Autodesk Inventor part; units mm, degrees
note: some values were not read from the file. Chosen so that the rebuilt part matches the saved one: direction of "Hole2".
(part 13 of 20)
  line L1144 (-97.751541, -32.701603) -> (-97.575214, -32.525276)
  line L1145 (-97.575214, -32.525276) -> (-96.427868, -32.525276)
  line L1146 (-96.251541, -32.701603) -> (-96.427868, -32.525276)
  line L1147 (-96.427868, -32.525276) -> (-96.427868, -31.87793)
  circle A26 centre (-97.263452, -32.201603) radius 0.1
  line L1148 (-97.101541, -32.351603) -> (-97.425364, -32.351603)
  line L1149 (-97.425364, -32.351603) -> (-97.425364, -32.051603)
  line L1150 (-97.425364, -32.051603) -> (-97.101541, -32.051603)
  line L1151 (-97.101541, -32.051603) -> (-97.101541, -32.351603)
  line L1152 (-98.151541, -33.912275) -> (-97.951541, -33.912275)
  line L1153 (-97.951541, -33.912275) -> (-97.951541, -34.160588)
  line L1154 (-98.151541, -33.912275) -> (-98.151541, -33.451603)
  line L1155 (-96.051541, -34.160588) -> (-97.951541, -34.160588)
  line L1156 (-95.851541, -33.451603) -> (-95.851541, -33.912275)
  line L1157 (-96.051541, -34.160588) -> (-96.051541, -33.912275)
  line L1158 (-96.051541, -33.912275) -> (-95.851541, -33.912275)
  line L1159 (-96.251541, -33.451603) -> (-96.251541, -33.912275)
  line L1160 (-96.251541, -33.912275) -> (-97.751541, -33.912275)
  line L1161 (-97.751541, -33.912275) -> (-97.751541, -33.451603)
  line L1162 (-97.575214, -33.451603) -> (-97.575214, -33.621159)
  line L1163 (-97.751541, -33.912275) -> (-97.575214, -33.621159)
  line L1164 (-97.575214, -33.621159) -> (-96.427868, -33.621159)
  line L1165 (-96.251541, -33.912275) -> (-96.427868, -33.621159)
  line L1166 (-96.427868, -33.621159) -> (-96.427868, -33.451603)
  line L1167 (-97.101541, -33.471854) -> (-97.425364, -33.471854)
  line L1168 (-97.425364, -33.471854) -> (-97.425364, -33.451603)
  line L1169 (-97.101541, -33.451603) -> (-97.101541, -33.471854)
  line L1170 (-105.474058, -21.298) -> (-105.497268, -21.496648)
  line L1171 (-105.474199, -21.298054) -> (-105.474058, -21.298)
  line L1172 (-105.745579, -21.467637) -> (-105.74572, -21.467691)
  line L1173 (-105.497268, -21.496648) -> (-105.745579, -21.467637)
  line L1174 (-105.713438, -23.585748) -> (-105.741108, -23.582515)
  line L1175 (-105.96621, -23.354854) -> (-105.74572, -21.467691)
  line L1176 (-105.474058, -21.298) -> (-105.214117, -21.32837)
  line L1177 (-104.271292, -21.775052) -> (-104.476203, -23.528871)
  line L1178 (-105.966068, -23.3548) -> (-105.745579, -21.467637)
  line L1179 (-104.747723, -23.698507) -> (-105.740967, -23.58246)
  line L1180 (-105.741108, -23.582515) -> (-105.729814, -23.485843)
  line L1181 (-105.745774, -23.380609) -> (-105.96621, -23.354854)
  line L1182 (-105.966068, -23.3548) -> (-105.717757, -23.383811)
  line L1183 (-105.717757, -23.383811) -> (-105.740967, -23.58246)
  line L1184 (-105.740967, -23.58246) -> (-105.741108, -23.582515)
  line L1185 (-105.717757, -23.383811) -> (-105.717899, -23.383866)
  line L1186 (-105.96621, -23.354854) -> (-105.966068, -23.3548)
  line L1187 (-104.476203, -23.528871) -> (-104.476344, -23.528925)
  line L1188 (-104.747723, -23.698507) -> (-104.724514, -23.499859)
  line L1189 (-104.724514, -23.499859) -> (-104.476203, -23.528871)
  line L1190 (-104.747864, -23.698562) -> (-104.747723, -23.698507)
  line L1191 (-104.527233, -21.811344) -> (-104.701304, -23.30121)
  line L1192 (-104.701304, -23.30121) -> (-105.694548, -23.185163)
  line L1193 (-105.694548, -23.185163) -> (-105.520477, -21.695297)
  line L1194 (-105.520477, -21.695297) -> (-104.527233, -21.811344)
  line L1195 (-104.856079, -23.105651) -> (-104.722932, -21.966057)
  line L1196 (-104.701304, -23.30121) -> (-104.856079, -23.105651)
  line L1197 (-104.527233, -21.811344) -> (-104.722932, -21.966057)
  line L1198 (-104.722932, -21.966057) -> (-105.365905, -21.890934)
  line L1199 (-105.520477, -21.695297) -> (-105.365905, -21.890934)
  line L1200 (-105.365905, -21.890934) -> (-105.499051, -23.030528)
  line L1201 (-105.694548, -23.185163) -> (-105.499051, -23.030528)
  line L1202 (-105.499051, -23.030528) -> (-104.856079, -23.105651)
  circle A27 centre (-105.080572, -22.238141) radius 0.1
  line L1203 (-105.248353, -22.381553) -> (-105.210775, -22.059918)
  line L1204 (-105.210795, -22.059926) -> (-105.210775, -22.059918)
  line L1205 (-105.248374, -22.381561) -> (-105.210795, -22.059926)
  line L1206 (-105.248374, -22.381561) -> (-105.248353, -22.381553)
  line L1207 (-105.210775, -22.059918) -> (-104.912801, -22.094733)
  line L1208 (-104.912801, -22.094733) -> (-104.95038, -22.416367)
  line L1209 (-104.9504, -22.416375) -> (-104.95038, -22.416367)
  line L1210 (-104.95038, -22.416367) -> (-105.248353, -22.381553)
  line L1211 (-104.9504, -22.416375) -> (-105.248374, -22.381561)
  line L1212 (-104.238991, -32.139646) -> (-104.43764, -32.116436)
  line L1213 (-104.238849, -32.139591) -> (-104.238991, -32.139646)
  line L1214 (-104.437498, -32.116382) -> (-104.238849, -32.139591)
  line L1215 (-104.43764, -32.116436) -> (-104.437498, -32.116382)
  line L1216 (-104.268003, -32.387957) -> (-104.238991, -32.139646)
  line L1217 (-104.267861, -32.387902) -> (-104.268003, -32.387957)
  line L1218 (-104.238849, -32.139591) -> (-104.267861, -32.387902)
  line L1219 (-104.122936, -31.146332) -> (-104.096258, -30.918)
  line L1220 (-104.321451, -31.123138) -> (-104.321593, -31.123193)
  line L1221 (-104.122802, -31.146348) -> (-104.321451, -31.123138)
  line L1222 (-104.09379, -30.898037) -> (-104.122802, -31.146348)
  line L1223 (-104.093932, -30.898091) -> (-104.09379, -30.898037)
  line L1224 (-104.43764, -32.116436) -> (-104.321593, -31.123193)
  line L1225 (-102.38084, -32.608447) -> (-104.268003, -32.387957)
  line L1226 (-104.437498, -32.116382) -> (-104.321451, -31.123138)
  line L1227 (-104.09379, -30.898037) -> (-102.206627, -31.118527)
  line L1228 (-102.380698, -32.608392) -> (-104.267861, -32.387902)
  line L1229 (-102.03699, -31.390047) -> (-102.153038, -32.383291)
  line L1230 (-102.153179, -32.383345) -> (-102.351695, -32.360151)
  line L1231 (-102.380698, -32.608392) -> (-102.351686, -32.360081)
  line L1232 (-102.351686, -32.360081) -> (-102.153038, -32.383291)
  line L1233 (-102.153038, -32.383291) -> (-102.153179, -32.383345)
  line L1234 (-102.38084, -32.608447) -> (-102.380698, -32.608392)
  line L1235 (-102.03699, -31.390047) -> (-102.235639, -31.366837)
  line L1236 (-102.235639, -31.366837) -> (-102.206627, -31.118527)
  line L1237 (-103.924153, -31.169557) -> (-102.434288, -31.343628)
  line L1238 (-102.434288, -31.343628) -> (-102.550335, -32.336872)
  line L1239 (-102.550335, -32.336872) -> (-104.040201, -32.162801)
  line L1240 (-104.040201, -32.162801) -> (-103.924153, -31.169557)
  line L1241 (-102.629987, -31.49834) -> (-103.769581, -31.365194)
  line L1242 (-102.434288, -31.343628) -> (-102.629987, -31.49834)
  line L1243 (-103.924153, -31.169557) -> (-103.769581, -31.365194)
  line L1244 (-103.769581, -31.365194) -> (-103.844704, -32.008166)
  line L1245 (-104.040201, -32.162801) -> (-103.844704, -32.008166)
  line L1246 (-103.844704, -32.008166) -> (-102.70511, -32.141313)
  line L1247 (-102.550335, -32.336872) -> (-102.70511, -32.141313)
  line L1248 (-102.70511, -32.141313) -> (-102.629987, -31.49834)
  circle A28 centre (-103.497462, -31.72285) radius 0.1
  line L1249 (-103.354057, -31.890627) -> (-103.675692, -31.853049)
  line L1250 (-103.675712, -31.853056) -> (-103.675692, -31.853049)
  line L1251 (-103.354077, -31.890635) -> (-103.675712, -31.853056)
  line L1252 (-103.354077, -31.890635) -> (-103.354057, -31.890627)
  line L1253 (-103.675692, -31.853049) -> (-103.640877, -31.555076)
  line L1254 (-103.640898, -31.555083) -> (-103.640877, -31.555076)
  line L1255 (-103.675712, -31.853056) -> (-103.640898, -31.555083)
  line L1256 (-103.640877, -31.555076) -> (-103.319243, -31.592654)
  line L1257 (-103.319243, -31.592654) -> (-103.354057, -31.890627)
  line L1258 (-100.436541, -20.036387) -> (-100.436541, -20.235039)
  line L1259 (-100.436541, -20.235039) -> (-100.686541, -20.235039)
  line L1260 (-99.436541, -20.235039) -> (-99.436541, -20.036387)
  line L1261 (-99.186541, -20.235039) -> (-99.436541, -20.235039)
  line L1262 (-99.186541, -22.284516) -> (-99.436541, -22.284516)
  line L1263 (-99.186541, -22.12223) -> (-99.186541, -22.284516)
  line L1264 (-99.436541, -22.320882) -> (-99.436541, -22.12223)
  line L1265 (-99.436541, -22.12223) -> (-99.186541, -22.12223)
  line L1266 (-99.436541, -22.483167) -> (-99.436541, -22.320882)
  line L1267 (-99.436541, -22.483167) -> (-100.436541, -22.483167)
  line L1268 (-100.436541, -20.036387) -> (-99.436541, -20.036387)
  line L1269 (-99.186541, -20.235039) -> (-99.186541, -22.12223)
  line L1270 (-100.686541, -22.12223) -> (-100.686541, -20.235039)
  line L1271 (-99.436541, -22.320882) -> (-100.436541, -22.320882)
  line L1272 (-100.436541, -22.284516) -> (-100.686541, -22.284516)
  line L1273 (-100.686541, -22.12223) -> (-100.436541, -22.12223)
  line L1274 (-100.436541, -22.12223) -> (-100.436541, -22.320882)
  line L1275 (-100.436541, -22.320882) -> (-100.436541, -22.483167)
  line L1276 (-100.686541, -22.284516) -> (-100.686541, -22.12223)
  line L1277 (-99.436541, -20.43369) -> (-99.436541, -21.923578)
  line L1278 (-99.436541, -21.923578) -> (-100.436541, -21.923578)
  line L1279 (-100.436541, -21.923578) -> (-100.436541, -20.43369)
  line L1280 (-100.436541, -20.43369) -> (-99.436541, -20.43369)
  line L1281 (-99.612868, -21.864358) -> (-99.612868, -20.724747)
  line L1282 (-99.436541, -21.923578) -> (-99.612868, -21.864358)
  line L1283 (-99.436541, -20.43369) -> (-99.612868, -20.724747)
  line L1284 (-99.612868, -20.724747) -> (-100.260214, -20.724747)
  line L1285 (-100.436541, -20.43369) -> (-100.260214, -20.724747)
  line L1286 (-100.260214, -20.724747) -> (-100.260214, -21.864358)
  line L1287 (-100.436541, -21.923578) -> (-100.260214, -21.864358)
  line L1288 (-100.260214, -21.864358) -> (-99.612868, -21.864358)
  ellipse E653 centre (-99.936541, -21.005427) end of major axis (-99.836541, -21.005427) minor radius 0.099326
  ellipse E654 centre (-99.936541, -21.011223) end of major axis (-99.836541, -21.011223) minor radius 0.099326 (-100.036541, -21.011223) -> (-99.836541, -21.011223) ccw
  line L1289 (-100.036541, -21.011223) -> (-100.036541, -21.005427)
  line L1290 (-99.836541, -21.011223) -> (-99.836541, -21.005427)
  line L1291 (-100.086541, -21.172043) -> (-100.086541, -20.850403)
  line L1292 (-100.086541, -21.195227) -> (-100.086541, -21.172043)
  line L1293 (-100.086541, -20.850403) -> (-99.786541, -20.850403)
  line L1294 (-99.786541, -20.850403) -> (-99.786541, -21.172043)
  line L1295 (-99.786541, -21.195227) -> (-99.786541, -21.172043)
  line L1296 (-99.786541, -21.172043) -> (-100.086541, -21.172043)
  line L1297 (-99.786541, -21.195227) -> (-100.086541, -21.195227)
  line L1298 (-97.951541, -30.752047) -> (-98.151541, -30.752047)
  line L1299 (-98.151541, -30.589761) -> (-97.951541, -30.589761)
  line L1300 (-98.151541, -30.752047) -> (-98.151541, -30.589761)
  line L1301 (-97.951541, -30.838076) -> (-97.951541, -31.000361)
  line L1302 (-97.951541, -30.589761) -> (-97.951541, -30.838076)
  line L1303 (-97.951541, -29.596502) -> (-98.151541, -29.596502)
  line L1304 (-97.951541, -29.348188) -> (-97.951541, -29.596502)
  line L1305 (-95.851541, -30.752047) -> (-96.051541, -30.752047)
  line L1306 (-96.051541, -30.838076) -> (-96.051541, -30.589761)
  line L1307 (-96.051541, -30.589761) -> (-95.851541, -30.589761)
  line L1308 (-95.851541, -30.589761) -> (-95.851541, -30.752047)
  line L1309 (-96.051541, -31.000361) -> (-96.051541, -30.838076)
  line L1310 (-96.051541, -31.000361) -> (-97.951541, -31.000361)
  line L1311 (-98.151541, -30.589761) -> (-98.151541, -29.596502)
  line L1312 (-97.951541, -29.348188) -> (-96.051541, -29.348188)
  line L1313 (-96.051541, -30.838076) -> (-97.951541, -30.838076)
  line L1314 (-95.851541, -29.596502) -> (-95.851541, -30.589761)
  line L1315 (-95.851541, -29.596502) -> (-96.051541, -29.596502)
  line L1316 (-96.051541, -29.596502) -> (-96.051541, -29.348188)
  line L1317 (-97.751541, -29.596502) -> (-96.251541, -29.596502)
  line L1318 (-96.251541, -29.596502) -> (-96.251541, -30.589761)
  line L1319 (-96.251541, -30.589761) -> (-97.751541, -30.589761)
  line L1320 (-97.751541, -30.589761) -> (-97.751541, -29.596502)
  line L1321 (-96.427868, -29.887559) -> (-97.575214, -29.887559)
  line L1322 (-96.251541, -29.596502) -> (-96.427868, -29.887559)
  line L1323 (-97.751541, -29.596502) -> (-97.575214, -29.887559)
  line L1324 (-97.575214, -29.887559) -> (-97.575214, -30.530541)
  line L1325 (-97.751541, -30.589761) -> (-97.575214, -30.530541)
  line L1326 (-97.575214, -30.530541) -> (-96.427868, -30.530541)
  line L1327 (-96.251541, -30.589761) -> (-96.427868, -30.530541)
  line L1328 (-96.427868, -30.530541) -> (-96.427868, -29.887559)
  ellipse E655 centre (-97.263452, -30.18007) end of major axis (-97.163452, -30.18007) minor radius 0.099326
  ellipse E656 centre (-97.263452, -30.185866) end of major axis (-97.163452, -30.185866) minor radius 0.099326 (-97.363452, -30.185866) -> (-97.163452, -30.185866) ccw
  line L1329 (-97.363452, -30.185866) -> (-97.363452, -30.18007)
  line L1330 (-97.163452, -30.185866) -> (-97.163452, -30.18007)
  line L1331 (-97.101541, -30.334855) -> (-97.425364, -30.334855)
  line L1332 (-97.425364, -30.358039) -> (-97.425364, -30.334855)
  line L1333 (-97.101541, -30.358039) -> (-97.425364, -30.358039)
  line L1334 (-97.101541, -30.358039) -> (-97.101541, -30.334855)
  line L1335 (-97.425364, -30.334855) -> (-97.425364, -30.036878)
  line L1336 (-97.425364, -30.036878) -> (-97.101541, -30.036878)
  line L1337 (-97.101541, -30.036878) -> (-97.101541, -30.334855)
  line L1338 (-91.651387, -32.360151) -> (-91.849903, -32.383345)
  line L1339 (-91.850044, -32.383291) -> (-91.651396, -32.360081)
  line L1340 (-91.849903, -32.383345) -> (-91.850044, -32.383291)
  line L1341 (-91.622384, -32.608392) -> (-91.622242, -32.608447)
  line L1342 (-91.651396, -32.360081) -> (-91.622384, -32.608392)
  line L1343 (-91.767443, -31.366837) -> (-91.966092, -31.390047)
  line L1344 (-91.796455, -31.118527) -> (-91.767443, -31.366837)
  line L1345 (-89.906824, -30.918) -> (-89.880146, -31.146332)
  line L1346 (-89.909292, -30.898037) -> (-89.90915, -30.898091)
  line L1347 (-89.681631, -31.123138) -> (-89.88028, -31.146348)
  line L1348 (-89.88028, -31.146348) -> (-89.909292, -30.898037)
  line L1349 (-89.68149, -31.123193) -> (-89.681631, -31.123138)
  line L1350 (-89.68149, -31.123193) -> (-89.565442, -32.116436)
  line L1351 (-89.735079, -32.387957) -> (-91.622242, -32.608447)
  line L1352 (-91.850044, -32.383291) -> (-91.966092, -31.390047)
  line L1353 (-91.796455, -31.118527) -> (-89.909292, -30.898037)
  line L1354 (-89.735221, -32.387902) -> (-91.622384, -32.608392)
  line L1355 (-89.681631, -31.123138) -> (-89.565584, -32.116382)
  line L1356 (-89.565442, -32.116436) -> (-89.764091, -32.139646)
  line L1357 (-89.764091, -32.139646) -> (-89.735079, -32.387957)
  line L1358 (-89.735221, -32.387902) -> (-89.764233, -32.139591)
  line L1359 (-89.764233, -32.139591) -> (-89.565584, -32.116382)
  line L1360 (-89.565584, -32.116382) -> (-89.565442, -32.116436)
  line L1361 (-89.764233, -32.139591) -> (-89.764091, -32.139646)
  line L1362 (-89.735079, -32.387957) -> (-89.735221, -32.387902)
  line L1363 (-91.568794, -31.343628) -> (-90.078929, -31.169557)
  line L1364 (-90.078929, -31.169557) -> (-89.962881, -32.162801)
  line L1365 (-89.962881, -32.162801) -> (-91.452747, -32.336872)
  line L1366 (-91.452747, -32.336872) -> (-91.568794, -31.343628)
  line L1367 (-90.233501, -31.365194) -> (-91.373095, -31.49834)
  line L1368 (-90.078929, -31.169557) -> (-90.233501, -31.365194)
  line L1369 (-91.568794, -31.343628) -> (-91.373095, -31.49834)
  line L1370 (-91.373095, -31.49834) -> (-91.297972, -32.141313)
  line L1371 (-91.452747, -32.336872) -> (-91.297972, -32.141313)
  line L1372 (-91.297972, -32.141313) -> (-90.158378, -32.008166)
  line L1373 (-89.962881, -32.162801) -> (-90.158378, -32.008166)
  line L1374 (-90.158378, -32.008166) -> (-90.233501, -31.365194)
  circle A29 centre (-91.025904, -31.783638) radius 0.1
  line L1375 (-90.847674, -31.913837) -> (-91.169309, -31.951416)
  line L1376 (-91.169289, -31.951423) -> (-91.169309, -31.951416)
  line L1377 (-90.847654, -31.913845) -> (-91.169289, -31.951423)
  line L1378 (-90.847654, -31.913845) -> (-90.847674, -31.913837)
  line L1379 (-91.169309, -31.951416) -> (-91.204123, -31.653442)
  line L1380 (-91.204123, -31.653442) -> (-90.882488, -31.615864)
  line L1381 (-90.882468, -31.615872) -> (-90.882488, -31.615864)
  line L1382 (-90.882488, -31.615864) -> (-90.847674, -31.913837)
  line L1383 (-90.882468, -31.615872) -> (-90.847654, -31.913845)
  line L1384 (-104.198228, -17.697968) -> (-104.179357, -17.498876)
  line L1385 (-104.179257, -17.49887) -> (-104.19813, -17.697977)
  line L1386 (-104.179357, -17.498876) -> (-104.179257, -17.49887)
  line L1387 (-104.447014, -17.674387) -> (-104.447114, -17.674393)
  line L1388 (-104.19813, -17.697977) -> (-104.447014, -17.674387)
  line L1389 (-103.202592, -17.792341) -> (-103.183719, -17.593233)
  line L1390 (-102.953707, -17.815931) -> (-103.202592, -17.792341)
  line L1391 (-104.467979, -17.894515) -> (-104.447114, -17.674393)
  line L1392 (-104.179257, -17.49887) -> (-103.183719, -17.593233)
  line L1393 (-102.953707, -17.815931) -> (-103.132997, -19.707453)
  line L1394 (-104.613112, -19.426734) -> (-104.447014, -17.674387)
  line L1395 (-103.400754, -19.88297) -> (-103.553192, -19.868521)
  line L1396 (-103.132997, -19.707453) -> (-103.133098, -19.707459)
  line L1397 (-103.400754, -19.88297) -> (-103.381882, -19.683863)
  line L1398 (-103.381882, -19.683863) -> (-103.132997, -19.707453)
  line L1399 (-103.400855, -19.882976) -> (-103.400754, -19.88297)
  line L1400 (-103.221464, -17.991448) -> (-103.363009, -19.484755)
  line L1401 (-103.363009, -19.484755) -> (-104.358547, -19.390392)
  line L1402 (-104.358547, -19.390392) -> (-104.217002, -17.897085)
  line L1403 (-104.217002, -17.897085) -> (-103.221464, -17.991448)
  line L1404 (-103.521982, -19.29258) -> (-103.413715, -18.150354)
  line L1405 (-103.363009, -19.484755) -> (-103.521982, -19.29258)
  line L1406 (-103.221464, -17.991448) -> (-103.413715, -18.150354)
  line L1407 (-103.413715, -18.150354) -> (-104.058172, -18.089268)
  line L1408 (-104.217002, -17.897085) -> (-104.058172, -18.089268)
  line L1409 (-104.058172, -18.089268) -> (-104.16644, -19.231495)
  line L1410 (-104.358547, -19.390392) -> (-104.16644, -19.231495)
  line L1411 (-104.16644, -19.231495) -> (-103.521982, -19.29258)
  circle A30 centre (-103.765345, -18.430181) radius 0.1
  line L1412 (-103.929957, -18.577215) -> (-103.8994, -18.254837)
  line L1413 (-103.929972, -18.577216) -> (-103.899415, -18.254838)
  line L1414 (-103.8994, -18.254837) -> (-103.600739, -18.283146)
  line L1415 (-103.600739, -18.283146) -> (-103.631296, -18.605524)
  line L1416 (-103.631296, -18.605524) -> (-103.929957, -18.577215)
  line L1417 (-102.707954, -28.310952) -> (-102.708054, -28.310958)
  line L1418 (-102.907062, -28.292079) -> (-102.707954, -28.310952)
  line L1419 (-102.907162, -28.292085) -> (-102.907062, -28.292079)
  line L1420 (-102.731545, -28.559836) -> (-102.731645, -28.559843)
  line L1421 (-102.707954, -28.310952) -> (-102.731545, -28.559836)
  line L1422 (-102.812699, -27.296541) -> (-102.812799, -27.296548)
  line L1423 (-102.613591, -27.315414) -> (-102.812699, -27.296541)
  line L1424 (-102.59, -27.06653) -> (-102.613591, -27.315414)
  line L1425 (-102.5901, -27.066536) -> (-102.59, -27.06653)
  line L1426 (-102.907062, -28.292079) -> (-102.812699, -27.296541)
  line L1427 (-102.59, -27.06653) -> (-100.698478, -27.24582)
  line L1428 (-100.840023, -28.739126) -> (-102.731545, -28.559836)
  line L1429 (-100.522962, -27.513577) -> (-100.617325, -28.509115)
  line L1430 (-100.840023, -28.739126) -> (-100.816432, -28.490242)
  line L1431 (-100.816432, -28.490242) -> (-100.617325, -28.509115)
  line L1432 (-100.617325, -28.509115) -> (-100.617425, -28.509121)
  line L1433 (-100.840123, -28.739133) -> (-100.840023, -28.739126)
  line L1434 (-100.522962, -27.513577) -> (-100.722069, -27.494704)
  line L1435 (-100.722069, -27.494704) -> (-100.698478, -27.24582)
  line L1436 (-102.414483, -27.334287) -> (-100.921177, -27.475831)
  line L1437 (-100.921177, -27.475831) -> (-101.01554, -28.471369)
  line L1438 (-101.01554, -28.471369) -> (-102.508847, -28.329825)
  line L1439 (-102.508847, -28.329825) -> (-102.414483, -27.334287)
  line L1440 (-101.113427, -27.634737) -> (-102.255654, -27.52647)
  line L1441 (-100.921177, -27.475831) -> (-101.113427, -27.634737)
  line L1442 (-102.414483, -27.334287) -> (-102.255654, -27.52647)
  line L1443 (-102.255654, -27.52647) -> (-102.316739, -28.170928)
  line L1444 (-102.508847, -28.329825) -> (-102.316739, -28.170928)
  line L1445 (-102.316739, -28.170928) -> (-101.174513, -28.279195)
  line L1446 (-101.01554, -28.471369) -> (-101.174513, -28.279195)
  line L1447 (-101.174513, -28.279195) -> (-101.113427, -27.634737)
  circle A31 centre (-101.975808, -27.878117) radius 0.1
  line L1448 (-101.828777, -28.042726) -> (-102.151155, -28.012169)
  line L1449 (-102.151155, -28.012169) -> (-102.122846, -27.713508)
  line L1450 (-102.151169, -28.01217) -> (-102.12286, -27.713508)
  line L1451 (-102.122846, -27.713508) -> (-101.800468, -27.744065)
  line L1452 (-101.800468, -27.744065) -> (-101.828777, -28.042726)
  line L1453 (-100.436541, -16.471901) -> (-100.436541, -16.671009)
  line L1454 (-100.436541, -16.671009) -> (-100.686541, -16.671009)
  line L1455 (-99.436541, -16.671009) -> (-99.436541, -16.471901)
  line L1456 (-99.186541, -16.671009) -> (-99.436541, -16.671009)
  line L1457 (-100.436541, -16.471901) -> (-99.436541, -16.471901)
  line L1458 (-99.186541, -16.671009) -> (-99.186541, -18.477093)
  line L1459 (-100.686541, -18.477093) -> (-100.686541, -16.671009)
  line L1460 (-99.436541, -16.870117) -> (-99.436541, -18.278179)
  line L1461 (-100.436541, -18.278179) -> (-100.436541, -16.870117)
  line L1462 (-100.436541, -16.870117) -> (-99.436541, -16.870117)
  line L1463 (-99.612868, -17.620683) -> (-99.612868, -17.139983)
  line L1464 (-99.436541, -16.870117) -> (-99.612868, -17.139983)
  line L1465 (-99.612868, -17.139983) -> (-100.260214, -17.139983)
  line L1466 (-100.436541, -16.870117) -> (-100.260214, -17.139983)
  line L1467 (-100.260214, -17.139983) -> (-100.260214, -17.620683)
  ellipse E657 centre (-99.936541, -17.426773) end of major axis (-99.836541, -17.426773) minor radius 0.099554
  ellipse E658 centre (-99.936541, -17.43149) end of major axis (-99.836541, -17.43149) minor radius 0.099554 (-100.036541, -17.43149) -> (-99.836541, -17.43149) ccw
  line L1468 (-100.036541, -17.43149) -> (-100.036541, -17.426773)
  line L1469 (-99.836541, -17.43149) -> (-99.836541, -17.426773)
  line L1470 (-100.086541, -17.592679) -> (-100.086541, -17.2703)
  line L1471 (-100.086541, -17.611544) -> (-100.086541, -17.592679)
  line L1472 (-100.086541, -17.2703) -> (-99.786541, -17.2703)
  line L1473 (-99.786541, -17.2703) -> (-99.786541, -17.592679)
  line L1474 (-99.786541, -17.611544) -> (-99.786541, -17.592679)
  line L1475 (-99.786541, -17.592679) -> (-100.086541, -17.592679)
  line L1476 (-99.786541, -17.611544) -> (-100.086541, -17.611544)
  line L1477 (-98.151541, -27.049529) -> (-97.951541, -27.049529)
  line L1478 (-98.151541, -27.080011) -> (-98.151541, -27.049529)
  line L1479 (-97.951541, -27.298414) -> (-97.951541, -27.328384)
  line L1480 (-97.951541, -27.049529) -> (-97.951541, -27.298414)
  line L1481 (-97.951541, -26.053987) -> (-98.151541, -26.053987)
  line L1482 (-97.951541, -25.805102) -> (-97.951541, -26.053987)
  line L1483 (-98.151541, -27.049529) -> (-98.151541, -26.053987)
  line L1484 (-97.951541, -25.805102) -> (-96.051541, -25.805102)
  line L1485 (-96.051541, -27.298414) -> (-97.951541, -27.298414)
  line L1486 (-95.851541, -26.053987) -> (-95.851541, -27.049529)
  line L1487 (-96.051541, -27.298414) -> (-96.051541, -27.049529)
  line L1488 (-96.051541, -27.049529) -> (-95.851541, -27.049529)
  line L1489 (-95.851541, -27.049529) -> (-95.851541, -27.080011)
  line L1490 (-96.051541, -27.328384) -> (-96.051541, -27.298414)
  line L1491 (-95.851541, -26.053987) -> (-96.051541, -26.053987)
  line L1492 (-96.051541, -26.053987) -> (-96.051541, -25.805102)
  line L1493 (-97.751541, -26.053987) -> (-96.251541, -26.053987)
  line L1494 (-96.251541, -26.053987) -> (-96.251541, -27.049529)
  line L1495 (-96.251541, -27.049529) -> (-97.751541, -27.049529)
  line L1496 (-97.751541, -27.049529) -> (-97.751541, -26.053987)
  line L1497 (-96.251541, -26.053987) -> (-96.31212, -26.146703)
  line L1498 (-97.751541, -26.053987) -> (-97.690962, -26.146703)
  line L1499 (-97.751541, -27.049529) -> (-97.69434, -27.023182)
  line L1500 (-96.251541, -27.049529) -> (-96.308742, -27.023182)
  line L1501 (-93.385757, -28.509115) -> (-93.18665, -28.490242)
  line L1502 (-93.385657, -28.509121) -> (-93.385757, -28.509115)
  line L1503 (-93.163059, -28.739126) -> (-93.162959, -28.739133)
  line L1504 (-93.18665, -28.490242) -> (-93.163059, -28.739126)
  line L1505 (-93.281013, -27.494704) -> (-93.480121, -27.513577)
  line L1506 (-93.304604, -27.24582) -> (-93.281013, -27.494704)
  line L1507 (-93.385757, -28.509115) -> (-93.480121, -27.513577)
  line L1508 (-93.304604, -27.24582) -> (-91.413082, -27.06653)
  line L1509 (-91.271537, -28.559836) -> (-93.163059, -28.739126)
  line L1510 (-91.190384, -27.296541) -> (-91.09602, -28.292079)
  line L1511 (-91.413082, -27.06653) -> (-91.412982, -27.066536)
  line L1512 (-91.190384, -27.296541) -> (-91.389491, -27.315414)
  line L1513 (-91.389491, -27.315414) -> (-91.413082, -27.06653)
  line L1514 (-91.190283, -27.296548) -> (-91.190384, -27.296541)
  line L1515 (-91.271537, -28.559836) -> (-91.295128, -28.310952)
  line L1516 (-91.295128, -28.310952) -> (-91.09602, -28.292079)
  line L1517 (-91.09602, -28.292079) -> (-91.09592, -28.292085)
  line L1518 (-91.295128, -28.310952) -> (-91.295028, -28.310958)
  line L1519 (-91.271437, -28.559843) -> (-91.271537, -28.559836)
  line L1520 (-93.081905, -27.475831) -> (-91.588599, -27.334287)
  line L1521 (-91.588599, -27.334287) -> (-91.494235, -28.329825)
  line L1522 (-91.494235, -28.329825) -> (-92.987542, -28.471369)
  line L1523 (-92.987542, -28.471369) -> (-93.081905, -27.475831)
  line L1524 (-91.747428, -27.52647) -> (-92.889655, -27.634737)
  line L1525 (-91.588599, -27.334287) -> (-91.747428, -27.52647)
  line L1526 (-93.081905, -27.475831) -> (-92.889655, -27.634737)
  line L1527 (-92.889655, -27.634737) -> (-92.828569, -28.279195)
  line L1528 (-92.987542, -28.471369) -> (-92.828569, -28.279195)
  line L1529 (-92.828569, -28.279195) -> (-91.686343, -28.170928)
  line L1530 (-91.494235, -28.329825) -> (-91.686343, -28.170928)
  line L1531 (-91.686343, -28.170928) -> (-91.747428, -27.52647)
  circle A32 centre (-92.548759, -27.927546) radius 0.1
  line L1532 (-92.373412, -28.061599) -> (-92.69579, -28.092155)
  line L1533 (-92.69579, -28.092155) -> (-92.724099, -27.793494)
  line L1534 (-92.724099, -27.793494) -> (-92.401721, -27.762937)
  line L1535 (-92.401721, -27.762937) -> (-92.373412, -28.061599)
  line L1536 (-92.401707, -27.762938) -> (-92.373398, -28.061599)
  line L1537 (-99.501541, -46.299561) -> (-99.501541, -46.099561)
  line L1538 (-99.501541, -46.099561) -> (-99.251541, -46.099561)
  line L1539 (-100.501541, -46.099561) -> (-100.501541, -46.299561)
  line L1540 (-100.751541, -46.099561) -> (-100.501541, -46.099561)
  line L1541 (-99.501541, -46.299561) -> (-100.501541, -46.299561)
  line L1542 (-100.751541, -46.099561) -> (-100.751541, -44.199561)
  line L1543 (-99.251541, -44.199561) -> (-99.251541, -46.099561)
  line L1544 (-100.501541, -43.999561) -> (-99.501541, -43.999561)
  line L1545 (-99.251541, -44.199561) -> (-99.501541, -44.199561)
  line L1546 (-99.501541, -44.199561) -> (-99.501541, -43.999561)
  line L1547 (-100.501541, -43.999561) -> (-100.501541, -44.199561)
  line L1548 (-100.501541, -44.199561) -> (-100.751541, -44.199561)
  line L1549 (-100.501541, -45.899561) -> (-100.501541, -44.399561)
  line L1550 (-100.501541, -44.399561) -> (-99.501541, -44.399561)
  line L1551 (-99.501541, -44.399561) -> (-99.501541, -45.899561)
  line L1552 (-99.501541, -45.899561) -> (-100.501541, -45.899561)
  line L1553 (-100.325214, -44.575888) -> (-100.325214, -45.723234)
  line L1554 (-100.501541, -44.399561) -> (-100.325214, -44.575888)
  line L1555 (-100.501541, -45.899561) -> (-100.325214, -45.723234)
  line L1556 (-100.325214, -45.723234) -> (-99.677868, -45.723234)
  line L1557 (-99.501541, -45.899561) -> (-99.677868, -45.723234)
  line L1558 (-99.677868, -45.723234) -> (-99.677868, -44.575888)
  line L1559 (-99.501541, -44.399561) -> (-99.677868, -44.575888)
  line L1560 (-99.677868, -44.575888) -> (-100.325214, -44.575888)
  circle A33 centre (-100.001541, -45.411473) radius 0.1
  line L1561 (-99.851541, -45.249561) -> (-99.851541, -45.573384)
  line L1562 (-99.851541, -45.573384) -> (-100.151541, -45.573384)
  line L1563 (-100.151541, -45.573384) -> (-100.151541, -45.249561)
  line L1564 (-100.151541, -45.249561) -> (-99.851541, -45.249561)
  line L1565 (-95.851541, -35.701561) -> (-96.051541, -35.701561)
  line L1566 (-96.051541, -35.701561) -> (-96.051541, -35.451561)
  line L1567 (-96.051541, -36.701561) -> (-95.851541, -36.701561)
  line L1568 (-96.051541, -36.951561) -> (-96.051541, -36.701561)
  line L1569 (-95.851541, -35.701561) -> (-95.851541, -36.701561)
  line L1570 (-96.051541, -36.951561) -> (-97.951541, -36.951561)
  line L1571 (-97.951541, -35.451561) -> (-96.051541, -35.451561)
  line L1572 (-98.151541, -36.701561) -> (-98.151541, -35.701561)
  line L1573 (-97.951541, -35.451561) -> (-97.951541, -35.701561)
  line L1574 (-97.951541, -35.701561) -> (-98.151541, -35.701561)
  line L1575 (-98.151541, -36.701561) -> (-97.951541, -36.701561)
  line L1576 (-97.951541, -36.701561) -> (-97.951541, -36.951561)
  line L1577 (-96.251541, -36.701561) -> (-97.751541, -36.701561)
  line L1578 (-97.751541, -36.701561) -> (-97.751541, -35.701561)
  line L1579 (-97.751541, -35.701561) -> (-96.251541, -35.701561)
  line L1580 (-96.251541, -35.701561) -> (-96.251541, -36.701561)
  line L1581 (-97.575214, -36.525234) -> (-96.427868, -36.525234)
  line L1582 (-97.751541, -36.701561) -> (-97.575214, -36.525234)
  line L1583 (-96.251541, -36.701561) -> (-96.427868, -36.525234)
  line L1584 (-96.427868, -36.525234) -> (-96.427868, -35.877888)
  line L1585 (-96.251541, -35.701561) -> (-96.427868, -35.877888)
  line L1586 (-96.427868, -35.877888) -> (-97.575214, -35.877888)
  line L1587 (-97.751541, -35.701561) -> (-97.575214, -35.877888)
  line L1588 (-97.575214, -35.877888) -> (-97.575214, -36.525234)
  circle A34 centre (-96.73963, -36.201561) radius 0.1
  line L1589 (-96.901541, -36.051561) -> (-96.577718, -36.051561)
  line L1590 (-96.577718, -36.051561) -> (-96.577718, -36.351561)
  line L1591 (-96.577718, -36.351561) -> (-96.901541, -36.351561)
  line L1592 (-96.901541, -36.351561) -> (-96.901541, -36.051561)
  line L1593 (-93.501541, -46.299561) -> (-93.501541, -46.099561)
  line L1594 (-93.501541, -46.099561) -> (-93.251541, -46.099561)
  line L1595 (-94.501541, -46.099561) -> (-94.501541, -46.299561)
  line L1596 (-94.751541, -46.099561) -> (-94.501541, -46.099561)
  line L1597 (-93.501541, -46.299561) -> (-94.501541, -46.299561)
  line L1598 (-94.751541, -46.099561) -> (-94.751541, -44.199561)
  line L1599 (-93.251541, -44.199561) -> (-93.251541, -46.099561)
  line L1600 (-94.501541, -43.999561) -> (-93.501541, -43.999561)
  line L1601 (-93.251541, -44.199561) -> (-93.501541, -44.199561)
  line L1602 (-93.501541, -44.199561) -> (-93.501541, -43.999561)
  line L1603 (-94.501541, -43.999561) -> (-94.501541, -44.199561)
  line L1604 (-94.501541, -44.199561) -> (-94.751541, -44.199561)
  line L1605 (-94.501541, -45.899561) -> (-94.501541, -44.399561)
  line L1606 (-94.501541, -44.399561) -> (-93.501541, -44.399561)
  line L1607 (-93.501541, -44.399561) -> (-93.501541, -45.899561)
  line L1608 (-93.501541, -45.899561) -> (-94.501541, -45.899561)
  line L1609 (-94.325214, -44.575888) -> (-94.325214, -45.723234)
  line L1610 (-94.501541, -44.399561) -> (-94.325214, -44.575888)
  line L1611 (-94.501541, -45.899561) -> (-94.325214, -45.723234)
  line L1612 (-94.325214, -45.723234) -> (-93.677868, -45.723234)
  line L1613 (-93.501541, -45.899561) -> (-93.677868, -45.723234)
  line L1614 (-93.677868, -45.723234) -> (-93.677868, -44.575888)
  line L1615 (-93.501541, -44.399561) -> (-93.677868, -44.575888)
  line L1616 (-93.677868, -44.575888) -> (-94.325214, -44.575888)
  circle A35 centre (-94.001541, -45.411473) radius 0.1
  line L1617 (-93.851541, -45.249561) -> (-93.851541, -45.573384)
  line L1618 (-93.851541, -45.573384) -> (-94.151541, -45.573384)
  line L1619 (-94.151541, -45.573384) -> (-94.151541, -45.249561)
  line L1620 (-94.151541, -45.249561) -> (-93.851541, -45.249561)
  line L1621 (-93.566541, -18.278179) -> (-93.566541, -18.477093)
  line L1622 (-93.566541, -18.477093) -> (-93.316541, -18.477093)
  line L1623 (-94.566541, -18.477093) -> (-94.566541, -18.278179)
  line L1624 (-94.816541, -18.477093) -> (-94.566541, -18.477093)
  line L1625 (-93.566541, -18.278179) -> (-94.566541, -18.278179)
  line L1626 (-94.816541, -18.477093) -> (-94.816541, -20.235039)
  line L1627 (-93.316541, -20.235039) -> (-93.316541, -18.477093)
  line L1628 (-94.566541, -18.676007) -> (-94.566541, -20.036387)
  line L1629 (-93.566541, -18.676007) -> (-94.566541, -18.676007)
  line L1630 (-93.566541, -20.036387) -> (-93.566541, -18.676007)
  line L1631 (-94.566541, -18.676007) -> (-94.40658, -18.929512)
  line L1632 (-93.566541, -18.676007) -> (-93.726502, -18.929512)
  ellipse E659 centre (-94.066541, -19.239499) end of major axis (-94.166541, -19.239499) minor radius 0.099457
  ellipse E660 centre (-94.066541, -19.244703) end of major axis (-94.166541, -19.244703) minor radius 0.099457 (-94.166541, -19.244703) -> (-93.966541, -19.244703) ccw
  line L1633 (-93.966541, -19.239499) -> (-93.966541, -19.244703)
  line L1634 (-94.166541, -19.239499) -> (-94.166541, -19.244703)
  line L1635 (-93.916541, -19.405735) -> (-93.916541, -19.083671)
  line L1636 (-93.916541, -19.416282) -> (-93.916541, -19.405735)
  line L1637 (-93.916541, -19.083671) -> (-94.216541, -19.083671)
  line L1638 (-94.216541, -19.083671) -> (-94.216541, -19.405735)
  line L1639 (-94.216541, -19.416282) -> (-94.216541, -19.405735)
  line L1640 (-94.216541, -19.405735) -> (-93.916541, -19.405735)
  line L1641 (-89.219892, -19.610031) -> (-89.240693, -19.411216)
  line L1642 (-89.240693, -19.411216) -> (-89.240921, -19.41114)
  line L1643 (-89.240921, -19.41114) -> (-89.22011, -19.610054)
  line L1644 (-89.22011, -19.610054) -> (-88.971467, -19.58404)
  line L1645 (-88.971467, -19.58404) -> (-88.971239, -19.584116)
  line L1646 (-90.214681, -19.714112) -> (-90.235493, -19.515198)
  line L1647 (-90.463324, -19.740127) -> (-90.214681, -19.714112)
  line L1648 (-88.788748, -21.328345) -> (-88.971239, -19.584116)
  line L1649 (-89.995932, -21.802788) -> (-89.731778, -21.77515)
  line L1650 (-89.240921, -19.41114) -> (-90.235493, -19.515198)
  line L1651 (-90.463324, -19.740127) -> (-90.265614, -21.629812)
  line L1652 (-89.99616, -21.802712) -> (-89.001588, -21.698654)
  line L1653 (-88.773757, -21.473725) -> (-88.971467, -19.58404)
  line L1654 (-90.265386, -21.629888) -> (-90.016961, -21.603896)
  line L1655 (-90.265614, -21.629812) -> (-90.265386, -21.629888)
  line L1656 (-90.016971, -21.603797) -> (-90.265614, -21.629812)
  line L1657 (-89.99616, -21.802712) -> (-90.016971, -21.603797)
  line L1658 (-89.995932, -21.802788) -> (-89.99616, -21.802712)
  line L1659 (-89.0224, -21.49974) -> (-89.001588, -21.698654)
  line L1660 (-88.773757, -21.473725) -> (-89.0224, -21.49974)
  line L1661 (-90.19387, -19.913026) -> (-90.037783, -21.404883)
  line L1662 (-89.199298, -19.808969) -> (-90.19387, -19.913026)
  line L1663 (-89.043212, -21.300825) -> (-89.199298, -19.808969)
  line L1664 (-90.037783, -21.404883) -> (-89.043212, -21.300825)
  line L1665 (-89.880598, -21.21122) -> (-89.999989, -20.070102)
  line L1666 (-90.19387, -19.913026) -> (-89.999989, -20.070102)
  line L1667 (-90.037783, -21.404883) -> (-89.880598, -21.21122)
  line L1668 (-89.999989, -20.070102) -> (-89.356157, -20.002741)
  line L1669 (-89.199298, -19.808969) -> (-89.356157, -20.002741)
  line L1670 (-89.356157, -20.002741) -> (-89.236767, -21.143858)
  line L1671 (-89.043212, -21.300825) -> (-89.236767, -21.143858)
  line L1672 (-89.236767, -21.143858) -> (-89.880598, -21.21122)
  circle A36 centre (-89.645672, -20.346477) radius 0.1
  line L1673 (-89.47963, -20.491903) -> (-89.513327, -20.169839)
  line L1674 (-89.479598, -20.491914) -> (-89.47963, -20.491903)
  line L1675 (-89.479598, -20.491914) -> (-89.513294, -20.16985)
  line L1676 (-89.513294, -20.16985) -> (-89.513327, -20.169839)
  line L1677 (-89.513327, -20.169839) -> (-89.811698, -20.201056)
  line L1678 (-89.811698, -20.201056) -> (-89.778002, -20.523121)
  line L1679 (-89.777969, -20.523132) -> (-89.778002, -20.523121)
  line L1680 (-89.778002, -20.523121) -> (-89.47963, -20.491903)
  line L1681 (-89.777969, -20.523132) -> (-89.479598, -20.491914)
  line L1682 (-93.566541, -20.036387) -> (-93.566541, -20.235039)
  line L1683 (-93.566541, -20.235039) -> (-93.316541, -20.235039)
  line L1684 (-94.566541, -20.235039) -> (-94.566541, -20.036387)
  line L1685 (-94.816541, -20.235039) -> (-94.566541, -20.235039)
  line L1686 (-93.566541, -22.284516) -> (-93.316541, -22.284516)
  line L1687 (-93.566541, -22.12223) -> (-93.566541, -22.320882)
  line L1688 (-93.316541, -22.12223) -> (-93.566541, -22.12223)
  line L1689 (-93.566541, -22.320882) -> (-93.566541, -22.483167)
  line L1690 (-93.316541, -22.284516) -> (-93.316541, -22.12223)
  line L1691 (-94.566541, -22.483167) -> (-93.566541, -22.483167)
  line L1692 (-93.566541, -20.036387) -> (-94.566541, -20.036387)
  line L1693 (-94.816541, -20.235039) -> (-94.816541, -22.12223)
  line L1694 (-94.566541, -22.320882) -> (-93.566541, -22.320882)
  line L1695 (-93.316541, -22.12223) -> (-93.316541, -20.235039)
  line L1696 (-94.816541, -22.284516) -> (-94.566541, -22.284516)
  line L1697 (-94.816541, -22.12223) -> (-94.816541, -22.284516)
  line L1698 (-94.566541, -22.12223) -> (-94.816541, -22.12223)
  line L1699 (-94.566541, -22.320882) -> (-94.566541, -22.12223)
  line L1700 (-94.566541, -22.483167) -> (-94.566541, -22.320882)
  line L1701 (-94.566541, -20.43369) -> (-94.566541, -21.923578)
  line L1702 (-93.566541, -20.43369) -> (-94.566541, -20.43369)
  line L1703 (-93.566541, -21.923578) -> (-93.566541, -20.43369)
  line L1704 (-94.566541, -21.923578) -> (-93.566541, -21.923578)
  line L1705 (-94.390214, -21.864358) -> (-94.390214, -20.724747)
  line L1706 (-94.566541, -20.43369) -> (-94.390214, -20.724747)
  line L1707 (-94.566541, -21.923578) -> (-94.390214, -21.864358)
  line L1708 (-94.390214, -20.724747) -> (-93.742868, -20.724747)
  line L1709 (-93.566541, -20.43369) -> (-93.742868, -20.724747)
  line L1710 (-93.742868, -20.724747) -> (-93.742868, -21.864358)
  line L1711 (-93.566541, -21.923578) -> (-93.742868, -21.864358)
  line L1712 (-93.742868, -21.864358) -> (-94.390214, -21.864358)
  ellipse E661 centre (-94.066541, -21.005427) end of major axis (-94.166541, -21.005427) minor radius 0.099326
  ellipse E662 centre (-94.066541, -21.011223) end of major axis (-94.166541, -21.011223) minor radius 0.099326 (-94.166541, -21.011223) -> (-93.966541, -21.011223) ccw
  line L1713 (-93.966541, -21.005427) -> (-93.966541, -21.011223)
  line L1714 (-94.166541, -21.005427) -> (-94.166541, -21.011223)
  line L1715 (-93.916541, -21.172043) -> (-93.916541, -20.850403)
  line L1716 (-93.916541, -21.195227) -> (-93.916541, -21.172043)
  line L1717 (-93.916541, -20.850403) -> (-94.216541, -20.850403)
  line L1718 (-94.216541, -20.850403) -> (-94.216541, -21.172043)
  line L1719 (-94.216541, -21.195227) -> (-94.216541, -21.172043)
  line L1720 (-94.216541, -21.172043) -> (-93.916541, -21.172043)
  line L1721 (-94.216541, -21.195227) -> (-93.916541, -21.195227)
  line L1722 (-88.528883, -21.298054) -> (-88.529024, -21.298)
  line L1723 (-88.529024, -21.298) -> (-88.505814, -21.496648)
  line L1724 (-88.505814, -21.496648) -> (-88.257504, -21.467637)
  line L1725 (-88.257504, -21.467637) -> (-88.257362, -21.467691)
  line L1726 (-88.036872, -23.354854) -> (-88.257362, -21.467691)
  line L1727 (-88.289644, -23.585748) -> (-88.261974, -23.582515)
  line L1728 (-88.529024, -21.298) -> (-88.788965, -21.32837)
  line L1729 (-89.73179, -21.775052) -> (-89.526879, -23.528871)
  line L1730 (-89.255359, -23.698507) -> (-88.262115, -23.58246)
  line L1731 (-88.037014, -23.3548) -> (-88.257504, -21.467637)
  line L1732 (-88.257308, -23.380609) -> (-88.036872, -23.354854)
  line L1733 (-88.261974, -23.582515) -> (-88.273269, -23.485843)
  line L1734 (-88.285325, -23.383811) -> (-88.262115, -23.58246)
  line L1735 (-88.037014, -23.3548) -> (-88.285325, -23.383811)
  line L1736 (-88.285325, -23.383811) -> (-88.285183, -23.383866)
  line L1737 (-88.262115, -23.58246) -> (-88.261974, -23.582515)
  line L1738 (-88.036872, -23.354854) -> (-88.037014, -23.3548)
  line L1739 (-89.526879, -23.528871) -> (-89.526738, -23.528925)
  line L1740 (-89.278568, -23.499859) -> (-89.526879, -23.528871)
  line L1741 (-89.255359, -23.698507) -> (-89.278568, -23.499859)
  line L1742 (-89.255218, -23.698562) -> (-89.255359, -23.698507)
  line L1743 (-89.475849, -21.811344) -> (-89.301778, -23.30121)
  line L1744 (-88.482605, -21.695297) -> (-89.475849, -21.811344)
  line L1745 (-88.308534, -23.185163) -> (-88.482605, -21.695297)
  line L1746 (-89.301778, -23.30121) -> (-88.308534, -23.185163)
  line L1747 (-89.147003, -23.105651) -> (-89.28015, -21.966057)
  line L1748 (-89.475849, -21.811344) -> (-89.28015, -21.966057)
  line L1749 (-89.301778, -23.30121) -> (-89.147003, -23.105651)
  line L1750 (-89.28015, -21.966057) -> (-88.637177, -21.890934)
  line L1751 (-88.482605, -21.695297) -> (-88.637177, -21.890934)
  line L1752 (-88.637177, -21.890934) -> (-88.504031, -23.030528)
  line L1753 (-88.308534, -23.185163) -> (-88.504031, -23.030528)
  line L1754 (-88.504031, -23.030528) -> (-89.147003, -23.105651)
  circle A37 centre (-88.92251, -22.238141) radius 0.1
  line L1755 (-88.754729, -22.381553) -> (-88.792307, -22.059918)
  line L1756 (-88.754709, -22.381561) -> (-88.754729, -22.381553)
  line L1757 (-88.754709, -22.381561) -> (-88.792287, -22.059926)
  line L1758 (-88.792287, -22.059926) -> (-88.792307, -22.059918)
  line L1759 (-88.792307, -22.059918) -> (-89.090281, -22.094733)
  line L1760 (-89.090281, -22.094733) -> (-89.052702, -22.416367)
  line L1761 (-89.052682, -22.416375) -> (-89.052702, -22.416367)
  line L1762 (-89.052702, -22.416367) -> (-88.754729, -22.381553)
  line L1763 (-89.052682, -22.416375) -> (-88.754709, -22.381561)
  line L1764 (-93.566541, -16.471901) -> (-93.566541, -16.671009)
  line L1765 (-93.566541, -16.671009) -> (-93.316541, -16.671009)
  line L1766 (-94.566541, -16.671009) -> (-94.566541, -16.471901)
  line L1767 (-94.816541, -16.671009) -> (-94.566541, -16.671009)
  line L1768 (-93.566541, -16.471901) -> (-94.566541, -16.471901)
  line L1769 (-94.816541, -16.671009) -> (-94.816541, -18.477093)
  line L1770 (-93.316541, -18.477093) -> (-93.316541, -16.671009)
  line L1771 (-94.566541, -16.870117) -> (-94.566541, -18.278179)
  line L1772 (-93.566541, -16.870117) -> (-94.566541, -16.870117)
  line L1773 (-93.566541, -18.278179) -> (-93.566541, -16.870117)
  line L1774 (-94.390214, -17.620683) -> (-94.390214, -17.139983)
  line L1775 (-94.566541, -16.870117) -> (-94.390214, -17.139983)
  line L1776 (-94.390214, -17.139983) -> (-93.742868, -17.139983)
  line L1777 (-93.566541, -16.870117) -> (-93.742868, -17.139983)
  line L1778 (-93.742868, -17.139983) -> (-93.742868, -17.620683)
  ellipse E663 centre (-94.066541, -17.426773) end of major axis (-94.166541, -17.426773) minor radius 0.099554
  ellipse E664 centre (-94.066541, -17.43149) end of major axis (-94.166541, -17.43149) minor radius 0.099554 (-94.166541, -17.43149) -> (-93.966541, -17.43149) ccw
  line L1779 (-93.966541, -17.426773) -> (-93.966541, -17.43149)
  line L1780 (-94.166541, -17.426773) -> (-94.166541, -17.43149)
  line L1781 (-93.916541, -17.592679) -> (-93.916541, -17.2703)
  line L1782 (-93.916541, -17.611544) -> (-93.916541, -17.592679)
  line L1783 (-93.916541, -17.2703) -> (-94.216541, -17.2703)
  line L1784 (-94.216541, -17.2703) -> (-94.216541, -17.592679)
  line L1785 (-94.216541, -17.611544) -> (-94.216541, -17.592679)
  line L1786 (-94.216541, -17.592679) -> (-93.916541, -17.592679)
  line L1787 (-94.216541, -17.611544) -> (-93.916541, -17.611544)
  line L1788 (-89.804854, -17.697968) -> (-89.823725, -17.498876)
  line L1789 (-89.823725, -17.498876) -> (-89.823825, -17.49887)
  line L1790 (-89.823825, -17.49887) -> (-89.804952, -17.697977)
  line L1791 (-89.804952, -17.697977) -> (-89.556068, -17.674387)
  line L1792 (-89.556068, -17.674387) -> (-89.555968, -17.674393)
  line L1793 (-90.80049, -17.792341) -> (-90.819363, -17.593233)
  line L1794 (-91.049375, -17.815931) -> (-90.80049, -17.792341)
  line L1795 (-89.535103, -17.894515) -> (-89.555968, -17.674393)
  line L1796 (-89.823825, -17.49887) -> (-90.819363, -17.593233)
  line L1797 (-91.049375, -17.815931) -> (-90.870085, -19.707453)
  line L1798 (-90.602328, -19.88297) -> (-90.449891, -19.868521)
  line L1799 (-89.38997, -19.426734) -> (-89.556068, -17.674387)
  line L1800 (-90.870085, -19.707453) -> (-90.869984, -19.707459)
  line L1801 (-90.6212, -19.683863) -> (-90.870085, -19.707453)
  line L1802 (-90.602328, -19.88297) -> (-90.6212, -19.683863)
  line L1803 (-90.602227, -19.882976) -> (-90.602328, -19.88297)
  line L1804 (-90.781618, -17.991448) -> (-90.640073, -19.484755)
  line L1805 (-89.78608, -17.897085) -> (-90.781618, -17.991448)
  line L1806 (-89.644535, -19.390392) -> (-89.78608, -17.897085)
  line L1807 (-90.640073, -19.484755) -> (-89.644535, -19.390392)
  line L1808 (-90.4811, -19.29258) -> (-90.589367, -18.150354)
  line L1809 (-90.781618, -17.991448) -> (-90.589367, -18.150354)
  line L1810 (-90.640073, -19.484755) -> (-90.4811, -19.29258)
  line L1811 (-90.589367, -18.150354) -> (-89.94491, -18.089268)
  line L1812 (-89.78608, -17.897085) -> (-89.94491, -18.089268)
  line L1813 (-89.94491, -18.089268) -> (-89.836642, -19.231495)
  line L1814 (-89.644535, -19.390392) -> (-89.836642, -19.231495)
  line L1815 (-89.836642, -19.231495) -> (-90.4811, -19.29258)
  circle A38 centre (-90.237737, -18.430181) radius 0.1
  line L1816 (-90.073125, -18.577215) -> (-90.103682, -18.254837)
  line L1817 (-90.07311, -18.577216) -> (-90.103667, -18.254838)
  line L1818 (-90.103682, -18.254837) -> (-90.402343, -18.283146)
  line L1819 (-90.402343, -18.283146) -> (-90.371786, -18.605524)
  line L1820 (-90.371786, -18.605524) -> (-90.073125, -18.577215)
  ellipse E665 centre (-107.527001, -21.571456) end of major axis (-108.72547, -21.632047) minor radius 0.214474 (-106.770374, -21.36789) -> (-108.703563, -21.669949) ccw
  ellipse E666 centre (-107.517065, -21.767985) end of major axis (-108.515789, -21.818477) minor radius 0.178729 (-106.985042, -21.590501) -> (-108.303339, -21.916811) ccw
  line L1821 (-108.497534, -21.850062) -> (-108.703563, -21.669949)
  ellipse E667 centre (-107.517065, -21.767985) end of major axis (-108.266108, -21.805854) minor radius 0.134046 (-107.241608, -21.629696) -> (-108.056514, -21.887503) ccw
  line L1822 (-108.72547, -21.632047) -> (-108.768367, -20.783546)
  ellipse E668 centre (-86.476082, -21.571456) end of major axis (-85.277612, -21.632047) minor radius 0.214474 (-85.299519, -21.669949) -> (-87.232708, -21.36789) ccw
  ellipse E669 centre (-86.486017, -21.767985) end of major axis (-85.487293, -21.818477) minor radius 0.178729 (-85.699743, -21.916811) -> (-87.01804, -21.590501) ccw
  line L1823 (-85.505548, -21.850062) -> (-85.299519, -21.669949)
  ellipse E670 centre (-86.486017, -21.767985) end of major axis (-85.736974, -21.805854) minor radius 0.134046 (-85.946568, -21.887503) -> (-86.761474, -21.629696) ccw
  line L1824 (-85.277612, -21.632047) -> (-85.234715, -20.783546)
  ellipse E671 centre (-97.001541, -6.884497) end of major axis (-97.567961, -6.884497) minor radius 0.563895 (-96.632568, -7.312337) -> (-97.370514, -7.312337) ccw
  line L1825 (-97.115144, -6.491672) -> (-96.716623, -6.59014)
  line L1826 (-96.716623, -6.59014) -> (-96.60302, -6.982964)
  line L1827 (-96.60302, -6.982964) -> (-96.864744, -7.253358)
  line L1828 (-97.116312, -7.220894) -> (-97.286459, -7.178853)
  line L1829 (-97.286459, -7.178853) -> (-97.400062, -6.786029)
  line L1830 (-97.400062, -6.786029) -> (-97.115144, -6.491672)
  line L1831 (-96.716623, -6.59014) -> (-96.716623, -6.679835)
  line L1832 (-97.115144, -6.580927) -> (-97.115144, -6.491672)